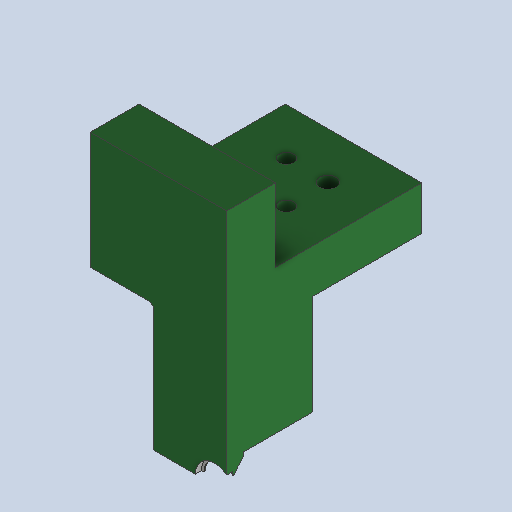
# Autodesk Inventor part: JH_int_Adapterplatte
Saved by Autodesk Inventor 2025.2 (Build 292293000, 293)
## iProperties
Created: 2025-06-17
Part Number: JH_int_Adapterplatte
Material: Generisch
Document SubType Name: Modeling
Designer: Jakob
Density: 1 g/cm^3
Appearance: Vorgabe
Author: Jakob
Autodesk Inventor part; units mm, degrees
ref_plane "YZ Plane" through (0, 0, 0) normal (1, 0, 0) x (0, 1, 0)
ref_plane "XZ Plane" through (0, 0, 0) normal (0, 1, 0) x (-1, 0, 0)
ref_plane "XY Plane" through (0, 0, 0) normal (0, 0, 1) x (1, 0, 0)
sketch "Skizze2" plane through (0, 0, 0) normal (0, 1, 0) x (-1, 0, 0)
  line L0 (14, 0) -> (-14, 0)
  line L1 (-14, 0) -> (-14, -5)
  line L2 (-14, -5) -> (1, -5)
  line L3 (1, -5) -> (1, -9)
  line L4 (1, -9) -> (14, -9)
  line L5 (14, -9) -> (14, 0)
  line L6 (0, -10.8) -> (0, 1.8) projected
  line L7 (19.6, 0) -> (-19.6, 0) projected
  point P0 (0, 0)
  dimension "d4" = 28
  dimension "d5" = 9
  dimension "d6" = 5
  dimension "d8" = 13
  dimension "d9" = 15
  constraints: 12 end point, 3 perpendicular, 2 horizontal, 1 collinear, 1 parallel, 1 other
  measures "d4" distance of L0.start L0.end
  measures "d5" distance of L4.end L0.start
  measures "d6" distance of L0.end L1.end
  measures "d8" distance of L3.end L4.end
  measures "d9" distance of L1.end L2.end
extrude "Extrusion2" add sketch "Skizze2" along normal blind 40
sketch "Skizze4" plane through (0, 40, 0) normal (0, 1, 0) x (1, 0, 0)
  line L0 (14, 5) -> (-1, 5)
  line L1 (-1, 5) -> (-1, 9)
  line L2 (-1, 9) -> (14, 9)
  line L3 (14, 9) -> (14, 5)
  line L4 (14, 5) -> (-1, 9) construction
  line L5 (-1, 5) -> (14, 9) construction
  line L6 (14, 5) -> (-1, 5) projected
  line L7 (-1, 5) -> (-1, 9) projected
  point P0 (0, 0)
  point P1 (6.5, 7)
  constraints: 12 end point, 4 collinear, 2 midpoint, 2 parallel, 1 horizontal, 1 perpendicular
extrude "Extrusion3" add sketch "Skizze4" against normal blind 22.5
sketch "Skizze6" plane through (14, 40, -9) normal (0, 0, -1) x (-1, 0, 0)
  line L0 (14, -48) -> (14, 8) projected
  line L1 (0, 0) -> (28, 0) projected
  point P0 (14, -40)
  point P1 (9.7574, -9.5074)
  point P2 (18.2426, -9.5074)
  point P3 (18.2426, -17.9926)
  point P4 (9.7574, -17.9926)
  dimension "d44" = 8.4853
  dimension "d45" = 8.4853
  dimension "d46" = 9.5074
  dimension "d47" = 17.9926
  constraints: 2 symmetric about line
  measures "d44" distance of point (18.243, -9.507) point (9.757, -9.507)
  measures "d45" distance of point (18.243, -17.993) point (9.757, -17.993)
  measures "d46" distance from line of L1 point (18.243, -9.507)
  measures "d47" distance from line of L1 point (18.243, -17.993)
hole "Bohrung3" at (4.2426, 22.0074, -9) at (-4.2426, 30.4926, -9) direction (0, 0, 1) diameter 3 end through all
hole "Bohrung4" at (4.2426, 30.4926, -9) at (-4.2426, 22.0074, -9) direction (0, 0, 1) diameter 3.4 end through all counterbore diameter 6.5 counterbore depth 3.4 clearance for "Sechskantkopfschraube DIN EN 24017" size "M3" standard "DIN"
sketch "Skizze8" plane through (-14, 0, 0) normal (0, 0, 1) x (1, 0, 0)
  line L0 (0, 0) -> (0, 40) projected
  line L1 (28, 0) -> (28, 17.5) projected
  line L2 (0, 0) -> (28, 0)
  line L3 (28, 0) -> (28, 10)
  line L4 (28, 10) -> (0, 10)
  line L5 (0, 10) -> (0, 0)
  point P0 (14, 0)
  point P1 (0, 10)
  dimension "d85" = 10
  constraints: 8 end point, 2 parallel, 1 horizontal, 1 perpendicular, 1 point on line
  measures "d85" distance between parallel lines of L2 L4
extrude "Extrusion4" add sketch "Skizze8" along normal blind 15
sketch "Skizze9" plane through (14, 0, -5) normal (0, 0, -1) x (-1, 0, 0)
  line L0 (0, 0) -> (15, 0) projected
  line L1 (15, 0) -> (15, 17.5) projected
  line L2 (0, 0) -> (15, 0)
  line L3 (15, 0) -> (15, 17.5)
  line L4 (15, 17.5) -> (0, 17.5)
  line L5 (0, 17.5) -> (0, 0)
  point P0 (14, 0)
  constraints: 8 end point, 2 parallel, 1 horizontal, 1 perpendicular
extrude "Extrusion5" add sketch "Skizze9" along normal blind 30
sketch "Skizze13" plane through (14, 0, -35) normal (0, 0, -1) x (-1, 0, 0)
  line L0 (0, 3.5) -> (0, 17.5) projected
  line L1 (15, 17.5) -> (0, 17.5) projected
  point P0 (14, 0)
  point P1 (11.95, 14.5)
  point P2 (11.95, 8.75)
  point P3 (6, 17.5)
  dimension "d102" = 11.95
  dimension "d103" = 3
  dimension "d104" = 8.75
  constraints: 1 vertical alignment
  measures "d102" distance from line of L0 point (11.95, 14.5)
  measures "d103" distance from line of L1 point (11.95, 14.5)
  measures "d104" distance from line of point (11.95, 8.75) L1
hole "Bohrung7" at (2.05, 14.5, -35) at (2.05, 8.75, -35) direction (0, 0, 1) diameter 4 depth 6 tip angle 118
sketch "Skizze14" plane through (-1, 0, -9) normal (-1, 0, 0) x (0, 0, 1)
  line L0 (0, 0) -> (-26, 0) projected
  line L1 (-26, 0) -> (-26, 17.5) projected
  point P0 (9, 0)
  point P1 (-20, 3)
  point P2 (-5.5, 3)
  dimension "d112" = 3
  dimension "d113" = 6
  dimension "d114" = 14.5
  constraints: 1 horizontal alignment
  measures "d112" distance from line of L0 point (-20, 3)
  measures "d113" distance from line of L1 point (-20, 3)
  measures "d114" distance of point (-5.5, 3) point (-20, 3)
hole "Bohrung8" at (-1, 3, -29) at (-1, 3, -14.5) direction (1, 0, 0) diameter 3.242 depth 8 tip angle 118 thread size "M4x0.7" class "6H" standard "ISO Metric profile"
fillet "Rundung2" radius 1 1 edges at (-1, 8.75, -9)
sketch "Skizze15" plane through (-1, 17.5, -35) normal (0, 1, 0) x (1, 0, 0)
  circle A0 centre (12.5, 0) radius 3.45
  line L0 (15, -26) -> (15, 0) projected
  line L1 (0, 0) -> (15, 0) projected
  point P0 (1, -35)
  dimension "d123" = 6.9
  dimension "d124" = 2.5
  constraints: 1 centre point, 1 point on line
  measures "d123" diameter of A0
  measures "d124" distance from line of L0 A0.centre
extrude "Extrusion9" cut sketch "Skizze15" against normal through all
sketch "Skizze16" plane through (-2, 17.5, -9) normal (0, 1, 0) x (1, 0, 0)
  circle A0 centre (13.5, 26) radius 6
  arc A1 (10.05, 26) -> (16, 23.6225) centre (13.5, 26) ccw projected
  point P0 (2, -9)
  dimension "d127" = 12
  constraints: 1 centre point, 1 concentric
  measures "d127" diameter of A0
extrude "Extrusion10" cut sketch "Skizze16" against normal blind 14
chamfer "Fasen3" distance 2 angle 45 1 edges at (10.2199, 3.5, -31.7963)
sketch "Skizze18" plane through (0, 0, 0) normal (0, -1, 0) x (1, 0, 0)
  circle A0 centre (11.5, -35) radius 3.95
  arc A1 (14, -32.6225) -> (8.05, -35) centre (11.5, -35) ccw projected
  point P0 (0, 0)
  dimension "d134" = 7.9
  constraints: 1 centre point, 1 concentric
  measures "d134" diameter of A0
extrude "Extrusion11" cut sketch "Skizze18" against normal blind 1.25
